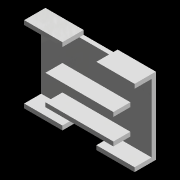
# Autodesk Inventor part: Belt Aligners
Saved by Autodesk Inventor 2014 SP1 (Build 180222100, 222)
## iProperties
Created: 2013-11-29
Part Number: Belt Aligners
Material: Polyethylene, High Density
Document SubType Name: Modeling
Designer: Rauhul Varma
Mass: 23.5226 g
Surface Area: 169.758 cm^2
Volume: 24.7086 cm^3
Density: 0.952 g/cm^3
Appearance: Smooth - Pure White
Author: Rauhul Varma
Autodesk Inventor part; units mm, degrees
ref_plane "YZ Plane" through (0, 0, 0) normal (1, 0, 0) x (0, 1, 0)
ref_plane "XZ Plane" through (0, 0, 0) normal (0, 1, 0) x (-1, 0, 0)
ref_plane "XY Plane" through (0, 0, 0) normal (0, 0, 1) x (1, 0, 0)
sketch "Sketch1" plane through (0, 0, 0) normal (0, 0, 1) x (1, 0, 0)
  line L0 (0, 0) -> (28.575, 0)
  line L1 (82.55, 0) -> (82.55, 57.15)
  line L2 (82.55, 57.15) -> (53.975, 57.15)
  line L3 (0, 57.15) -> (0, 0)
  line L4 (0, 53.975) -> (28.575, 53.975) construction
  line L5 (28.575, 57.15) -> (28.575, 53.975)
  line L6 (53.975, 57.15) -> (53.975, 53.975)
  line L7 (53.975, 53.975) -> (82.55, 53.975) construction
  line L8 (28.575, 53.975) -> (53.975, 53.975)
  line L9 (53.975, 57.15) -> (28.575, 57.15) construction
  line L10 (28.575, 57.15) -> (0, 57.15)
  line L11 (0, 3.175) -> (28.575, 3.175) construction
  line L12 (53.975, 0) -> (53.975, 3.175)
  line L13 (28.575, 0) -> (28.575, 3.175)
  line L14 (28.575, 0) -> (53.975, 0) construction
  line L15 (53.975, 0) -> (82.55, 0)
  line L16 (53.975, 3.175) -> (82.55, 3.175) construction
  line L17 (28.575, 3.175) -> (53.975, 3.175)
  dimension "d0" = 82.55
  dimension "d1" = 57.15
  dimension "d2" = 28.575
  dimension "d3" = 25.4
  dimension "d4" = 3.175
  dimension "d5" = 3.175
  dimension "d6" = 28.575
  dimension "d7" = 25.4
  constraints: 36 end point, 15 perpendicular, 12 parallel, 6 point on line, 3 horizontal
  measures "d0" distance of L3.start L1.end
  measures "d1" distance of L1.end L1.start
  measures "d2" distance between parallel lines of L3 L5
  measures "d3" distance between parallel lines of L6 L5
  measures "d4" distance of L5.start L4.end
  measures "d5" distance of L12.start L12.end
  measures "d6" distance between parallel lines of L3 L13
  measures "d7" distance between parallel lines of L12 L13
extrude "Extrusion1" add sketch "Sketch1" along normal blind 3.175
sketch "Sketch4" plane through (0, 0, 3.175) normal (0, 0, 1) x (1, 0, 0)
  line L0 (82.55, 0) -> (82.55, 57.15) projected
  line L1 (53.975, 53.975) -> (28.575, 53.975) projected
  line L2 (0, 57.15) -> (0, 0) projected
  line L3 (28.575, 3.175) -> (53.975, 3.175) projected
  line L4 (28.575, 3.175) -> (0, 3.175)
  line L5 (0, 3.175) -> (0, 0)
  line L6 (0, 0) -> (28.575, 0)
  line L7 (28.575, 0) -> (28.575, 3.175)
  line L8 (53.975, 3.175) -> (82.55, 3.175)
  line L9 (82.55, 3.175) -> (82.55, 0)
  line L10 (82.55, 0) -> (53.975, 0)
  line L11 (53.975, 0) -> (53.975, 3.175)
  line L12 (53.975, 53.975) -> (82.55, 53.975)
  line L13 (82.55, 53.975) -> (82.55, 57.15)
  line L14 (82.55, 57.15) -> (53.975, 57.15)
  line L15 (53.975, 57.15) -> (53.975, 53.975)
  line L16 (28.575, 53.975) -> (0, 53.975)
  line L17 (0, 53.975) -> (0, 57.15)
  line L18 (0, 57.15) -> (28.575, 57.15)
  line L19 (28.575, 57.15) -> (28.575, 53.975)
  line L20 (0, 28.575) -> (82.55, 28.575) construction
  line L21 (41.275, 53.975) -> (41.275, 3.175) construction
  line L22 (23.775, 47.2281) -> (58.775, 47.2281) construction
  line L23 (58.775, 47.2281) -> (58.775, 9.9219) construction
  line L24 (58.775, 9.9219) -> (23.775, 9.9219) construction
  line L25 (23.775, 9.9219) -> (23.775, 47.2281) construction
  line L26 (0, 27.3573) -> (82.55, 27.3573) construction
  line L27 (82.55, 12.3573) -> (0, 12.3573) construction
  line L28 (6.35, 8.7312) -> (76.2, 8.7312)
  line L29 (76.2, 8.7312) -> (76.2, 11.9062)
  line L30 (76.2, 11.9062) -> (6.35, 11.9062)
  line L31 (6.35, 11.9062) -> (6.35, 8.7312)
  line L32 (0, 19.8573) -> (82.55, 19.8573) construction
  line L33 (76.2, 27.8083) -> (76.2, 30.9833)
  line L34 (76.2, 30.9833) -> (6.35, 30.9833)
  line L35 (6.35, 30.9833) -> (6.35, 27.8083)
  line L36 (6.35, 27.8083) -> (76.2, 27.8083)
  dimension "d39" = 35
  dimension "d40" = 37.3062
  dimension "d41" = 15
  dimension "d42" = 2.4354
  dimension "d43" = 69.85
  dimension "d44" = 3.175
  dimension "d45" = 5.5563
  dimension "d46" = 0.451
  dimension "d47" = 69.85
  constraints: 66 end point, 13 parallel, 13 perpendicular, 6 point on line, 5 horizontal, 4 midpoint, 7 other
  measures "d39" distance of L23.end L24.end
  measures "d40" distance between parallel lines of L22 L24
  measures "d41" distance between parallel lines of L26 L27
  measures "d42" distance between parallel lines of L27 L24
  measures "d43" distance of L28.start L28.end
  measures "d44" distance between parallel lines of L30 L28
  measures "d45" distance between parallel lines of L3 L28
  measures "d46" distance between parallel lines of L27 L30
  measures "d47" distance of L33.end L34.end
extrude "Extrusion4" add sketch "Sketch4" along normal blind 12.7 contours L10 L11 L8 L0 | L12 L15 L14 L0 | L7 L6 L2 L4 | L16 L2 L18 L19 | L31 L30 L29 L28 | L36 L35 L34 L33
equation "\"d2\" = -0.5 * d3 + 0.5 * d0"
equation "\"d6\" = d2"
equation "\"d7\" = d3"
equation "\"d42\" = -0.666667 * d41 + 0.333333 * d40"
equation "\"d43\" = d47"
body "Solid1"
